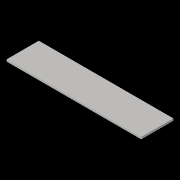
# Autodesk Inventor part: NLNMNMNR
Saved by Autodesk Inventor 2016 (Build 200138000, 138)
## iProperties
Created: 2017-01-21
Part Number: NLNMNMNR
Material: Generic
Document SubType Name: Modeling
Designer: Alexis Renderos
Density: 1 g/cm^3
Appearance: Default
Author: Alexis Renderos
Autodesk Inventor part; units mm, degrees
ref_plane "YZ Plane" through (0, 0, 0) normal (1, 0, 0) x (0, 1, 0)
ref_plane "XZ Plane" through (0, 0, 0) normal (0, 1, 0) x (-1, 0, 0)
ref_plane "XY Plane" through (0, 0, 0) normal (0, 0, 1) x (1, 0, 0)
sketch "Sketch1" plane through (0, 0, 0) normal (0, 1, 0) x (-1, 0, 0)
  line L0 (0, -71.12) -> (0, 71.12) projected
  line L1 (-299.3085, 0) -> (299.3085, 0) projected
  line L2 (213.7918, 50.8) -> (-213.7918, 50.8)
  line L3 (-213.7918, 50.8) -> (-213.7918, -50.8)
  line L4 (-213.7918, -50.8) -> (213.7918, -50.8)
  line L5 (213.7918, -50.8) -> (213.7918, 50.8)
  line L6 (213.7918, 50.8) -> (-213.7918, -50.8) construction
  line L7 (-213.7918, 50.8) -> (213.7918, -50.8) construction
  point P0 (0, 0)
  dimension "d0" = 427.5836
  dimension "d1" = 101.6
  constraints: 12 end point, 2 midpoint, 2 parallel, 1 horizontal, 1 perpendicular
  measures "d0" distance of L4.end L3.end
  measures "d1" distance of L3.end L2.end
extrude "Extrusion1" add sketch "Sketch1" along normal mid plane 6.35
body "Solid1"
